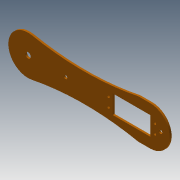
# Autodesk Inventor part: dibond_strana(b)
Saved by Autodesk Inventor 2013 (Build 170138000, 138)
## iProperties
Created: 2013-05-10
Part Number: dibond_strana(b)
Material: Generic
Document SubType Name: Modeling
Designer: idle-rug
Density: 1 g/cm^3
Author: idle-rug
Autodesk Inventor part; units mm, degrees
ref_plane "YZ Plane" through (0, 0, 0) normal (1, 0, 0) x (0, 1, 0)
ref_plane "XZ Plane" through (0, 0, 0) normal (0, 1, 0) x (-1, 0, 0)
ref_plane "XY Plane" through (0, 0, 0) normal (0, 0, 1) x (1, 0, 0)
sketch "Sketch1" plane through (0, 0, 0) normal (0, 1, 0) x (-1, 0, 0)
  line L0 (60, 0) -> (70.5, 0)
  circle A0 centre (70.5, 0) radius 21
  line L1 (60, 21) -> (70.5, 21)
  line L2 (60, -21) -> (70.5, -21)
  line L3 (-60, 0) -> (-70.5, 0)
  circle A1 centre (-70.5, 0) radius 21
  line L4 (-60, 21) -> (-70.5, 21)
  line L5 (-60, -21) -> (-70.5, -21)
  arc A2 (-55.8816, 20.5922) -> (55.8816, 20.5922) centre (0, 300) ccw
  arc A3 (55.8816, -20.5922) -> (-55.8816, -20.5922) centre (0, -300) ccw
  arc A4 (-57.1726, 20.8535) -> (0, 15.0588) centre (0, 300) ccw
  arc A5 (57.8833, -21) -> (-57.8833, -21) centre (0, -300) ccw
  line L6 (-60, -21) -> (-57.8833, -21)
  line L7 (70.5, -21) -> (57.8833, -21)
  arc A6 (-57.8833, 21) -> (57.8833, 21) centre (0, 300) ccw
  line L8 (-70.5, 21) -> (-57.8833, 21)
  line L9 (70.5, 21) -> (57.8833, 21)
  dimension "d3" = 42
  dimension "d5" = 42
  constraints: 20 end point, 17 point on circle, 7 centre point, 6 tangent, 3 coincident, 2 collinear, 2 parallel
  measures "d3" diameter of A0
  measures "d5" diameter of A1
extrude "Extrusion1" add sketch "Sketch1" along normal blind 2
sketch "Sketch3" plane through (0, 2, 0) normal (0, 1, 0) x (1, 0, 0)
  arc A0 (-70.5, 21) -> (-70.5, -21) centre (-70.5, 0) ccw projected
  line L0 (-70.5, -21) -> (-57.8833, -21) projected
  line L1 (-57.8833, 21) -> (-70.5, 21) projected
  line L2 (-70.5, 0) -> (-60, 0)
  arc A1 (-70.5, 21) -> (-70.5, -21) centre (-70.5, 0) ccw
  arc A2 (-60, 21) -> (-60, -21) centre (-60, 0) ccw
  line L3 (-70.5, 21) -> (-60, 21)
  line L4 (-70.5, -21) -> (-60, -21)
  point P0 (0, 0)
  dimension "d27" = 10.5
  constraints: 7 tangent, 6 end point, 4 point on circle, 2 centre point, 2 collinear, 2 point on line, 1 parallel
  measures "d27" distance of L2.start L2.end
extrude "Extrusion2" cut sketch "Sketch3" against normal blind 2
sketch "Sketch4" plane through (0, 2, 0) normal (0, 1, 0) x (1, 0, 0)
  arc A0 (-60, 21) -> (-60, -21) centre (-60, 0) ccw projected
  arc A1 (70.5, -21) -> (70.5, 21) centre (70.5, 0) ccw projected
  line L0 (-57.8833, 21) -> (-60, 21) projected
  circle A2 centre (-60, 0) radius 3
  line L1 (70.5, 0) -> (60, 0)
  circle A3 centre (60, 0) radius 3
  line L2 (-60, 0) -> (-20, 0)
  circle A4 centre (-20, 0) radius 2
  point P0 (0, 0)
  dimension "d30" = 6
  dimension "d31" = 10.5
  dimension "d32" = 6
  dimension "d33" = 40
  dimension "d34" = 4
  constraints: 4 end point, 3 centre point, 3 coincident, 1 collinear, 1 parallel
  measures "d30" diameter of A2
  measures "d31" distance of L1.start L1.end
  measures "d32" diameter of A3
  measures "d33" distance of L2.start L2.end
  measures "d34" diameter of A4
extrude "Extrusion3" cut sketch "Sketch4" against normal blind 2
sketch "Sketch5" plane through (0, 2, 0) normal (0, 1, 0) x (1, 0, 0)
  arc A0 (-60, 21) -> (-60, -21) centre (-60, 0) ccw projected
  line L0 (-60, -21) -> (-57.8833, -21) projected
  arc A1 (57.8833, -21) -> (-57.8833, -21) centre (0, -300) ccw projected
  arc A2 (-57.8833, 21) -> (57.8833, 21) centre (0, 300) ccw projected
  circle A3 centre (-60, 0) radius 21
  line L1 (-60, -21) -> (-57.8833, -21)
  line L2 (-55.8816, -20.5922) -> (-57.8833, -21)
  line L3 (-55.8816, -20.5922) -> (-55.8816, 20.5922)
  line L4 (-55.8816, -21.5122) -> (-81.7819, -21.5122)
  line L5 (-81.7819, -21.5122) -> (-81.7819, 22.1513)
  line L6 (-81.7819, 22.1513) -> (-55.8816, 22.1513)
  line L7 (-55.8816, 22.1513) -> (-55.8816, -21.5122)
  point P0 (0, 0)
  constraints: 14 end point, 5 point on circle, 2 parallel, 1 centre point, 1 coincident, 1 horizontal, 1 perpendicular, 1 point on line, 1 tangent
extrude "Extrusion4" cut sketch "Sketch5" against normal blind 2 contours A3 L3 A0 | A0 L0 A1 L7 L4 L5 L6 A3 | A3 A1 L0
sketch "Sketch6" plane through (0, 2, 0) normal (0, 1, 0) x (1, 0, 0)
  line L0 (70.5, 21) -> (57.8833, 21) projected
  circle A0 centre (-20, 0) radius 2 projected
  line L1 (-20, 0) -> (-60, 0)
  circle A1 centre (-60, 0) radius 21
  circle A2 centre (-60, 0) radius 3
  point P0 (0, 0)
  dimension "d39" = 40
  dimension "d40" = 6
  constraints: 2 centre point, 2 coincident, 2 end point, 1 parallel
  measures "d39" distance of L1.start L1.end
  measures "d40" diameter of A2
extrude "Extrusion5" cut sketch "Sketch6" against normal blind 2 contours A1
sketch "Sketch7" plane through (0, 2, 0) normal (0, 1, 0) x (1, 0, 0)
  arc A0 (-55.8816, -20.5922) -> (-55.8816, 20.5922) centre (-60, 0) ccw projected
  circle A1 centre (-60, 0) radius 21
  circle A2 centre (-60, 0) radius 3
  point P0 (0, 0)
  dimension "d43" = 6
  constraints: 2 coincident, 1 centre point, 3 other
  measures "d43" diameter of A2
extrude "Extrusion6" add sketch "Sketch7" against normal blind 2
sketch "Sketch8" plane through (0, 2, 0) normal (0, 1, 0) x (1, 0, 0)
  circle A0 centre (-60, 0) radius 3 projected
  circle A1 centre (60, 0) radius 3 projected
  circle A2 centre (-20, 0) radius 2 projected
  point P0 (0, 0)
extrude "Extrusion7" add sketch "Sketch8" against normal blind 2
sketch "Sketch9" plane through (0, 2, 0) normal (0, 1, 0) x (1, 0, 0)
  arc A0 (70.5, -21) -> (70.5, 21) centre (70.5, 0) ccw projected
  line L0 (70.5, 21) -> (57.8833, 21) projected
  line L1 (70.5, 0) -> (60, 0)
  line L2 (60, 0) -> (78.1, 0)
  line L3 (78.1, 0) -> (23.1, 0)
  line L4 (23.1, 0) -> (50.6, 0)
  line L5 (78.1, 10) -> (23.1, 10)
  line L6 (23.1, 10) -> (23.1, -10)
  line L7 (23.1, -10) -> (78.1, -10)
  line L8 (78.1, -10) -> (78.1, 10)
  line L9 (78.1, 10) -> (23.1, -10) construction
  line L10 (23.1, 10) -> (78.1, -10) construction
  line L11 (70.7, 10) -> (30.5, 10)
  line L12 (30.5, 10) -> (30.5, -10)
  line L13 (30.5, -10) -> (70.7, -10)
  line L14 (70.7, -10) -> (70.7, 10)
  line L15 (70.7, 10) -> (30.5, -10) construction
  line L16 (30.5, 10) -> (70.7, -10) construction
  line L17 (30.5, 0) -> (26.8, 0)
  line L18 (26.8, 0) -> (26.8, 4.95)
  line L19 (26.8, 0) -> (26.8, -4.95)
  line L20 (23.1, 4.95) -> (25.75, 4.95)
  line L21 (23.1, -4.95) -> (25.75, -4.95)
  circle A1 centre (25.75, -4.95) radius 1.5
  circle A2 centre (25.75, 4.95) radius 1.5
  line L22 (23.1, 4.95) -> (78.1, 4.95)
  line L23 (23.1, -4.95) -> (78.1, -4.95)
  line L24 (78.1, 4.95) -> (75.45, 4.95)
  line L25 (78.1, -4.95) -> (75.45, -4.95)
  circle A3 centre (75.45, 4.95) radius 1.5
  circle A4 centre (75.45, -4.95) radius 1.5
  point P0 (0, 0)
  dimension "d48" = 10.5
  dimension "d49" = 18.1
  dimension "d50" = 55
  dimension "d51" = 27.5
  dimension "d52" = 20
  dimension "d53" = 40.2
  dimension "d54" = 3.7
  dimension "d56" = 2.65
  dimension "d57" = 2.65
  dimension "d58" = 3
  dimension "d59" = 3
  dimension "d60" = 2.65
  dimension "d61" = 2.65
  dimension "d62" = 3
  dimension "d63" = 3
  constraints: 50 end point, 9 point on line, 6 midpoint, 6 parallel, 5 coincident, 5 perpendicular, 4 centre point, 2 collinear, 2 horizontal
  measures "d48" distance of L1.start L1.end
  measures "d49" distance of L1.end L2.end
  measures "d50" distance of L2.end L3.end
  measures "d51" distance of L3.end L4.end
  measures "d52" distance of L6.end L5.end
  measures "d53" distance of L13.end L12.end
  measures "d54" distance of L17.start L17.end
  measures "d56" distance of L20.start L20.end
  measures "d57" distance of L21.start L21.end
  measures "d58" diameter of A1
  measures "d59" diameter of A2
  measures "d60" distance of L22.end L24.end
  measures "d61" distance of L23.end L25.end
  measures "d62" diameter of A3
  measures "d63" diameter of A4
extrude "Extrusion8" cut sketch "Sketch9" against normal blind 2 contours L2 L14 L23 L12 L3 L1 | L1 L3 L12 L22 L14 L2 | L14 L7 L12 L23 | L22 L12 L5 L14 | A4 L23 | L23 A4 | A3 L22 | L22 A3 | L23 L19 A1 | A1 L21 L23 | L22 L20 A2 | A2 L18 L22 | A2 L20 L22 L18 | L19 L23 L21 A1
sketch "Sketch10" plane through (0, 2, 0) normal (0, 1, 0) x (1, 0, 0)
  arc A0 (-55.8816, 20.5922) -> (-55.8816, -20.5922) centre (-60, 0) ccw projected
  arc A1 (70.5, -21) -> (70.5, 21) centre (70.5, 0) ccw projected
  line L0 (70.5, 21) -> (57.8833, 21) projected
  circle A2 centre (-60, 0) radius 3
  line L1 (-60, 0) -> (-20, 0)
  line L2 (91.5, 0) -> (81.5, 0)
  circle A3 centre (-20, 0) radius 2
  circle A4 centre (81.5, 0) radius 2
  point P0 (0, 0)
  dimension "d66" = 6
  dimension "d67" = 40
  dimension "d69" = 10
  dimension "d71" = 4
  dimension "d72" = 4
  constraints: 4 end point, 3 centre point, 2 coincident, 1 collinear, 1 parallel, 1 point on circle
  measures "d66" diameter of A2
  measures "d67" distance of L1.start L1.end
  measures "d69" distance of L2.start L2.end
  measures "d71" diameter of A3
  measures "d72" diameter of A4
extrude "Extrusion9" cut sketch "Sketch10" against normal blind 2
body "Solid1"
